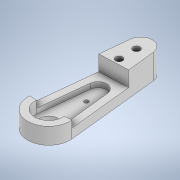
# Autodesk Inventor part: servoarm
Saved by Autodesk Inventor 2020.3 (Build 243373000, 373)
## iProperties
Created: 2021-03-19
Part Number: servoarm
Material: Generic
Document SubType Name: Modeling
Designer: 0x6f736f646f
Density: 1 g/cm^3
Appearance: Default
Author: 0x6f736f646f
Autodesk Inventor part; units mm, degrees
ref_plane "YZ Plane" through (0, 0, 0) normal (1, 0, 0) x (0, 1, 0)
ref_plane "XZ Plane" through (0, 0, 0) normal (0, 1, 0) x (-1, 0, 0)
ref_plane "XY Plane" through (0, 0, 0) normal (0, 0, 1) x (1, 0, 0)
sketch "Sketch1" plane through (0, 0, 0) normal (0, 1, 0) x (-1, 0, 0)
  circle A0 centre (-7.5, 4.5) radius 1
  circle A1 centre (-7.5, 9.5) radius 1
  circle A2 centre (-7.5, 18.84) radius 0.6
  circle A3 centre (-7.5, 29.5) radius 2.5
  circle A4 centre (-7.5, 29.576) radius 6.0215
  circle A5 centre (-7.5, 29.576) radius 4.0045
  circle A6 centre (-7.5, 3.274) radius 3.274
  circle A7 centre (-7.5, 15.5) radius 2.5045
  line L0 (-7.5, 3.274) -> (-7.5, 29.576)
  line L1 (-3.5183, 29.1493) -> (-5.0098, 15.2331)
  line L2 (-9.9902, 15.2331) -> (-11.4817, 29.1493)
  line L3 (-1.5114, 28.947) -> (-4.2439, 2.932)
  line L4 (-13.4886, 28.947) -> (-10.7561, 2.932)
  line L5 (-1.5114, 28.947) -> (-3.5183, 29.1493)
  line L6 (-13.4886, 28.947) -> (-11.4817, 29.1493)
  line L7 (-3.4324, 10.6581) -> (-11.5347, 10.3447)
  line L8 (-3.3796, 11.1605) -> (-11.587, 10.843)
  point P0 (0, 0)
  point P1 (-7.5, 10.5007)
  point P2 (-7.5, 10.5)
  point P3 (-7.5387, 10.4993)
  dimension "d2" = 2
  dimension "d3" = 2
  dimension "d4" = 1.2
  dimension "d5" = 5
  dimension "d6" = 12.043
  dimension "d7" = 8.009
  dimension "d8" = 6.548
  dimension "d9" = 5.009
  dimension "d10" = 5
  dimension "d11" = 1.226
  dimension "d12" = 6
  dimension "d15" = 26.302
  dimension "d16" = 3.34
  dimension "d17" = 10.66
  dimension "d18" = 26.302
  dimension "d19" = 25
  dimension "d28" = 0.5
  constraints: 18 end point, 9 point on circle, 9 tangent, 8 centre point, 4 point on line, 1 concentric, 1 parallel, 1 vertical
  measures "d2" diameter of A0
  measures "d3" diameter of A1
  measures "d4" diameter of A2
  measures "d5" diameter of A3
  measures "d6" diameter of A4
  measures "d7" diameter of A5
  measures "d8" diameter of A6
  measures "d9" diameter of A7
  measures "d10" distance of A0.centre A1.centre
  measures "d11" distance of L0.start A0.centre
  measures "d12" distance of A1.centre A7.centre
  measures "d15" distance of A4.centre L0.start
  measures "d16" distance of A7.centre A2.centre
  measures "d17" distance of A3.centre A2.centre
  measures "d18" distance of L0.start L0.end
  measures "d19" distance of A3.centre A0.centre
  measures "d28" distance between parallel lines of L7 L8
extrude "Extrusion1" add sketch "Sketch1" along normal blind 4.7 contours A4 L5 A5 L6
extrude "Extrusion2" add sketch "Sketch1" along normal blind 2.7 contours A6 | A6 L4 L7 A1 L0 | L0 A1 L7 L3 A6 | L4 L8 L0 L7 | L0 L8 L3 L7 | L4 A4 L2 A7 L0 L8 | L0 A7 L1 A4 L3 L8 | L6 L2 A4 | A4 L1 L5
extrude "Extrusion3" add sketch "Sketch1" along normal blind 1.2 contours L0 A7 | A7 L0 | L2 A5 L0 A4 | A4 L0 A2 A7 L2 | A5 | A7 L0 A2 A4 L1 | A4 L0 A5 L1
extrude "Extrusion4" add sketch "Sketch1" along normal blind 7.1 contours A6 | A6 L4 L7 A1 L0 | L0 A1 L7 L3 A6 | L4 L8 L0 L7 | L0 L8 L3 L7
body "Solid1"
